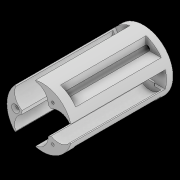
# Autodesk Inventor part: akkuhalterung_2
Saved by Autodesk Inventor 2022 (Build 260153000, 153)
## iProperties
Created: 2021-04-19
Part Number: akkuhalterung_2
Material: Generisch
Document SubType Name: Modeling
Designer: g.schardt
Density: 1 g/cm^3
Appearance: Vorgabe
Author: g.schardt
Autodesk Inventor part; units mm, degrees
ref_plane "YZ Plane" through (0, 0, 0) normal (1, 0, 0) x (0, 1, 0)
sketch "Skizze1" plane through (0, 0, 0) normal (0, 0, 1) x (1, 0, 0)
  circle A0 centre (0, 0) radius 20.25
  dimension "d0" = 40.5
  constraints: 1 centre point, 1 coincident
  measures "d0" diameter of A0
extrude "Extrusion1" add sketch "Skizze1" along normal blind 8
sketch "Skizze2" plane through (0, 0, 8) normal (0, 0, 1) x (1, 0, 0)
  circle A0 centre (11, 0) radius 9.5
  circle A1 centre (0, 0) radius 20.25 projected
  circle A2 centre (-5.5, 9.5263) radius 9.5
  circle A3 centre (-5.5, -9.5263) radius 9.5
  point P0 (1.5, 0)
  point P1 (-0.75, 1.299)
  point P2 (-0.75, -1.299)
  dimension "d3" = 19
  dimension "d6" = 360
  dimension "d251" = 40.5
  dimension "d252" = 11
  constraints: 3 horizontal alignment, 18 other
  measures "d251" diameter of A1
  measures "d252" distance of point (11, 0) A1.centre
extrude "Extrusion2" cut sketch "Skizze2" against normal blind 4.5 contours A0 A1 | A1 A0 | A2 A1 | A1 A2 | A3 A1 | A1 A3
sketch "Skizze3" plane through (-5.5, 9.5263, 8) normal (0, 0, 1) x (-0.8660254, -0.5, 0)
  circle A0 centre (0, 11) radius 10
  dimension "d10" = 20
  constraints: 1 centre point, 1 coincident
  measures "d10" diameter of A0
extrude "Extrusion3" cut sketch "Skizze3" against normal blind 4.5
sketch "Skizze4" plane through (0, 0, 3.5) normal (0, 0, 1) x (1, 0, 0)
  line L0 (5, 5.75) -> (25, 5.75)
  line L1 (25, 5.75) -> (25, -5.75)
  line L2 (25, -5.75) -> (5, -5.75)
  line L3 (5, -5.75) -> (5, 5.75)
  circle A0 centre (0, 0) radius 20.25 projected
  arc A1 (5.9432, -8.0423) -> (5.9432, 8.0423) centre (11, 0) ccw projected
  arc A2 (5.9432, 8.0423) -> (3.9932, 9.1681) centre (0, 0) ccw projected
  arc A3 (5.9432, -8.0423) -> (20.0369, -2.9298) centre (11, 0) ccw projected
  arc A4 (-7.4812, -18.8174) -> (20.0369, -2.9298) centre (0, 0) ccw projected
  arc A5 (3.9932, 9.1681) -> (-7.4812, 18.8174) centre (-5.5, 9.5263) ccw projected
  arc A6 (3.9932, -9.1681) -> (5.9432, -8.0423) centre (0, 0) ccw projected
  arc A7 (-9.9364, -1.1258) -> (-12.5558, -15.8876) centre (-5.5, -9.5263) ccw projected
  arc A8 (-9.9364, 1.1258) -> (-9.9364, -1.1258) centre (0, 0) ccw projected
  arc A9 (-12.5558, 15.8876) -> (-12.5558, -15.8876) centre (0, 0) ccw projected
  arc A10 (20.0369, 2.9298) -> (5.9432, 8.0423) centre (11, 0) ccw projected
  arc A11 (-12.5558, 15.8876) -> (-9.9364, 1.1258) centre (-5.5, 9.5263) ccw projected
  arc A12 (20.0369, 2.9298) -> (-7.4812, 18.8174) centre (0, 0) ccw projected
  arc A13 (-7.4812, -18.8174) -> (3.9932, -9.1681) centre (-5.5, -9.5263) ccw projected
  point P0 (25, 0)
  point P1 (20.25, 0)
  point P2 (19.4165, 5.75)
  point P3 (18.5622, 5.75)
  point P4 (19.4165, -5.75)
  point P5 (18.5622, -5.75)
  dimension "d13" = 20
  dimension "d14" = 11.5
  dimension "d33" = 6
  constraints: 8 end point, 2 parallel, 1 horizontal, 1 horizontal alignment, 1 midpoint, 1 perpendicular, 1 other
  measures "d13" distance of L1.end L2.end
  measures "d14" distance of L0.end L1.end
  measures "d33" distance from line of L3 A1.centre
extrude "Extrusion4" cut sketch "Skizze4" against normal blind 2 contours L0 A1 A0 L2 L3 | L0 A0 A1 | L0 L1 L2 A0 A1 | A1 A0 | A1 A0 L2
sketch "Skizze25" plane through (0, 0, 8) normal (0, 0, 1) x (1, 0, 0)
  arc A0 (19.4165, -5.75) -> (19.4165, 5.75) centre (0, 0) ccw projected
  line L0 (5, 5.75) -> (19.4165, 5.75) projected
  line L1 (5, -5.75) -> (5, 5.75) projected
  line L2 (19.4165, -5.75) -> (5, -5.75) projected
extrude "Extrusion21" cut sketch "Skizze25" against normal blind 4.5
sketch "Skizze6" plane through (0, 0, 3.5) normal (0, 0, 1) x (1, 0, 0)
  line L0 (5, 5.75) -> (14, 5.75)
  line L1 (14, 3.95) -> (5, 3.95)
  line L2 (5, 3.95) -> (5, 5.75)
  line L3 (18.5622, -5.75) -> (5, -5.75) projected
  line L4 (5, -5.75) -> (14, -5.75)
  line L5 (14, -3.95) -> (5, -3.95)
  line L6 (5, -3.95) -> (5, -5.75)
  line L7 (14, 3.95) -> (14, 5.75)
  line L8 (5, 5.75) -> (18.5622, 5.75) projected
  line L9 (14, -3.95) -> (14, -5.75)
  point P0 (0, 0)
  point P1 (19.4165, 5.75)
  point P2 (8.1815, -5.75)
  point P3 (8.1815, -5.75)
  dimension "d238" = 1.8
  dimension "d239" = 1.8
  dimension "d240" = 9
  dimension "d242" = 9
  constraints: 16 end point, 3 parallel, 2 horizontal, 2 perpendicular, 1 point on line
  measures "d238" distance of L1.end L0.start
  measures "d239" distance of L5.end L3.end
  measures "d240" distance of L1.start L1.end
  measures "d242" distance of L5.start L5.end
extrude "Extrusion6" add sketch "Skizze6" against normal blind 1.3
pattern_circular "Runde Anordnung1" count 3 over 360 about axis through (0, 0, 0) along (0, 0, 1) of "Extrusion4", "Extrusion6", "Extrusion21"
sketch "Skizze7" plane through (0, 0, 3.5) normal (0, 0, 1) x (1, 0, 0)
  circle A0 centre (0, 0) radius 5.5
  dimension "d40" = 11
  constraints: 1 centre point, 1 coincident
  measures "d40" diameter of A0
extrude "Extrusion7" cut sketch "Skizze7" against normal blind 2
sketch "Skizze26" plane through (0, 0, 8) normal (0, 0, 1) x (1, 0, 0)
  line L0 (-4.7286, 19.6902) -> (-4.3015, 18.9504) projected
  arc A0 (3.9932, 9.1681) -> (-4.3015, 18.9504) centre (-5.5, 9.5263) ccw projected
  arc A1 (5.9432, 8.0423) -> (3.9932, 9.1681) centre (0, 0) ccw projected
  arc A2 (18.5622, 5.75) -> (5.9432, 8.0423) centre (11, 0) ccw projected
  line L1 (18.5622, 5.75) -> (19.4165, 5.75) projected
  arc A3 (19.4165, 5.75) -> (-4.7286, 19.6902) centre (0, 0) ccw projected
  line L2 (-4.3015, -18.9504) -> (-4.7286, -19.6902) projected
  arc A4 (-4.7286, -19.6902) -> (19.4165, -5.75) centre (0, 0) ccw projected
  line L3 (19.4165, -5.75) -> (18.5622, -5.75) projected
  arc A5 (5.9432, -8.0423) -> (18.5622, -5.75) centre (11, 0) ccw projected
  arc A6 (3.9932, -9.1681) -> (5.9432, -8.0423) centre (0, 0) ccw projected
  arc A7 (-4.3015, -18.9504) -> (3.9932, -9.1681) centre (-5.5, -9.5263) ccw projected
  line L4 (-14.6879, -13.9402) -> (-14.2608, -13.2004) projected
  arc A8 (-9.9364, -1.1258) -> (-14.2608, -13.2004) centre (-5.5, -9.5263) ccw projected
  arc A9 (-9.9364, 1.1258) -> (-9.9364, -1.1258) centre (0, 0) ccw projected
  arc A10 (-14.2608, 13.2004) -> (-9.9364, 1.1258) centre (-5.5, 9.5263) ccw projected
  line L5 (-14.2608, 13.2004) -> (-14.6879, 13.9402) projected
  arc A11 (-14.6879, 13.9402) -> (-14.6879, -13.9402) centre (0, 0) ccw projected
extrude "Extrusion22" add sketch "Skizze26" along normal blind 58
sketch "Skizze28" plane through (0, 0, 0) normal (0, 0, -1) x (-1, 0, 0)
  circle A0 centre (0, 0) radius 14.8
  circle A1 centre (0, 0) radius 13.5
  dimension "d134" = 29.6
  dimension "d135" = 27
  constraints: 2 centre point, 2 coincident
  measures "d134" diameter of A0
  measures "d135" diameter of A1
extrude "Extrusion23" [suppressed]
sketch "Skizze29" plane through (0, 0, 66) normal (0, 0, 1) x (1, 0, 0)
  point P0 (0, 0)
  point P1 (-14.5, 0)
  dimension "d138" = 14.5
  constraints: 1 horizontal alignment
  measures "d138" distance of point (-14.5, 0) point (0, 0)
hole "Bohrung4" at (-14.5, 0, 66) direction (0, 0, -1) diameter 2.3 end through all
sketch "Skizze41" plane through (0, 0, 66) normal (0, 0, 1) x (1, 0, 0)
  circle A0 centre (-0.1, -0.1732) radius 2.5 construction
  circle A1 centre (-14.6, -0.1732) radius 1.75 construction
  circle A2 centre (-0.1, -0.1732) radius 14.5 construction
  line L0 (-0.1, -0.1732) -> (10.125, 17.537) construction
  circle A3 centre (0, 0) radius 20.25 construction
  line L1 (-0.1, -0.1732) -> (20.35, -0.1732) construction
  point P0 (7.15, 12.3842)
  dimension "d184" = 60
  constraints: 4 end point, 2 point on circle, 1 centre point, 1 coincident, 1 equal length, 1 horizontal, 1 point on line, 2 other
  measures "d184" angle of L1 L0
hole "Bohrung7" at (7.15, 12.3842, 66) direction (0, 0, -1) diameter 1.8 end through all
sketch "Skizze43" plane through (0, 0, 0) normal (0, 0, -1) x (-1, 0, 0)
  arc A0 (-8.0493, 12.4197) -> (-6.7311, 13.1807) centre (-7.15, 12.3842) ccw projected
  point P0 (0, 0)
hole "Bohrung8" at (7.15, 12.3842, 0) direction (0, 0, 1) diameter 3.5 depth 60 tip angle 118
pattern_circular "Runde Anordnung6" count 2 over 240 about axis through (0, 0, 0) along (0, 0, 1) of "Bohrung7", "Bohrung8"
sketch "Skizze44" plane through (0, 0, 0) normal (0, 0, -1) x (-1, 0, 0)
  circle A0 centre (0, 0) radius 20.25 projected
  circle A1 centre (0, 0) radius 18.25
  dimension "d202" = 2
  constraints: 1 centre point
  measures "d202" radial gap between concentric circles of A0 A1
extrude "Extrusion31" add sketch "Skizze44" along normal blind 3
sketch "Skizze45" plane through (0, 0, 1.5) normal (0, 0, 1) x (1, 0, 0)
  line L0 (0, 0) -> (-5, 8.6603) construction
  line L1 (0, 0) -> (10, 0) construction
  line L2 (0.9208, 6.3051) -> (-0.5157, 5.4758) construction
  point P0 (-1.25, 2.1651)
  dimension "d207" = 10
  dimension "d208" = 120
  dimension "d209" = 2.5
  constraints: 4 end point, 1 equal length, 1 horizontal, 1 point on line
  measures "d207" distance of L0.start L0.end
  measures "d208" angle of L1 L0
  measures "d209" distance from line of point (-1.25, 2.165) L2
hole "Bohrung9" at (-1.25, 2.1651, 1.5) direction (0, 0, -1) diameter 5 depth 80
sketch "Skizze46" plane through (0, 0, 66) normal (0, 0, 1) x (1, 0, 0)
  circle A0 centre (-14.5, 0) radius 1.15 projected
  arc A1 (-9.9364, 1.1258) -> (-9.9364, -1.1258) centre (0, 0) ccw projected
  arc A2 (-14.2608, 13.2004) -> (-9.9364, 1.1258) centre (-5.5, 9.5263) ccw projected
  line L0 (-14.2608, 13.2004) -> (-14.6879, 13.9402) projected
  arc A3 (-14.6879, 13.9402) -> (-14.6879, -13.9402) centre (0, 0) ccw projected
  line L1 (-14.6879, -13.9402) -> (-14.2608, -13.2004) projected
  arc A4 (-9.9364, -1.1258) -> (-14.2608, -13.2004) centre (-5.5, -9.5263) ccw projected
extrude "Extrusion32" add sketch "Skizze46" along normal blind 4
chamfer "Fase2" distance 1.5 angle 45 1 edges at (-15.65, 0, 70)
sketch "Skizze47" plane through (0, 0, 0) normal (0, 0, -1) x (-1, 0, 0)
  circle A0 centre (14.5, 0) radius 1.15 projected
  point P0 (0, 0)
hole "Bohrung10" at (-14.5, 0, 0) direction (0, 0, 1) diameter 3.5 depth 60 tip angle 118
ref_plane "Arbeitsebene4" through (0, 0, 60) normal (0, 0, 1) x (1, 0, 0)
sketch "Skizze48" plane through (0, 0, 60) normal (0, 0, 1) x (1, 0, 0)
  line L0 (6.25, 11.4842) -> (16.6786, 11.4842)
  line L1 (16.6786, 11.4842) -> (16.6786, 19.2614)
  line L2 (16.6786, 19.2614) -> (6.25, 19.2614)
  line L3 (6.25, 19.2614) -> (6.25, 11.4842)
  circle A0 centre (7.15, 12.3842) radius 0.9 projected
  circle A1 centre (0, 0) radius 20.25 projected
  point P0 (6.25, 12.3842)
  point P1 (7.15, 11.4842)
  constraints: 8 end point, 2 parallel, 2 point on circle, 2 tangent, 1 horizontal, 1 perpendicular
extrude "Extrusion33" cut sketch "Skizze48" against normal blind 58.5 contours A0 L3 A1 L0
ref_plane "Arbeitsebene5" through (0, 0, 60) normal (0, 0, 1) x (1, 0, 0)
sketch "Skizze49" plane through (0, 0, 60) normal (0, 0, 1) x (1, 0, 0)
  circle A0 centre (7.15, -12.3842) radius 0.9 projected
  line L0 (6.25, -11.4842) -> (16.6786, -11.4842)
  line L1 (16.6786, -11.4842) -> (16.6786, -19.2614)
  line L2 (16.6786, -19.2614) -> (6.25, -19.2614)
  line L3 (6.25, -19.2614) -> (6.25, -11.4842)
  arc A1 (-4.7286, -19.6902) -> (19.4165, -5.75) centre (0, 0) ccw projected
  point P0 (7.15, -11.4842)
  point P1 (6.25, -12.3842)
  constraints: 8 end point, 2 parallel, 2 point on circle, 2 tangent, 1 horizontal, 1 perpendicular
extrude "Extrusion34" cut sketch "Skizze49" against normal blind 58.5 contours A0 L0 A1 L3
chamfer "Fase3" distance 1 angle 45 6 edges at (14, 4.85, 2.2) (14, -4.85, 2.2) (-11.2002, -9.6994, 2.2) (-2.7998, -14.5494, 2.2) (-2.7998, 14.5494, 2.2) (-11.2002, 9.6994, 2.2)
sketch "Skizze39" plane through (0, 0, 66) normal (0, 0, 1) x (1, 0, 0)
  circle A0 centre (0, 0) radius 20.4
  constraints: 1 centre point, 1 coincident
sketch "Skizze31" plane through (0, 0, 66) normal (0, 0, 1) x (1, 0, 0)
  line L0 (-20.25, -5.5) -> (-17.25, -5.5)
  line L1 (-17.25, -5.5) -> (-17.25, 5.5)
  line L2 (-17.25, 5.5) -> (-20.25, 5.5)
  line L3 (-20.25, 5.5) -> (-20.25, -5.5)
  arc A0 (-14.6879, 13.9402) -> (-14.6879, -13.9402) centre (0, 0) ccw projected
  point P0 (-17.25, 0)
  point P1 (-19.6446, 5.5)
  point P2 (-19.6446, -5.5)
  dimension "d153" = 3
  dimension "d154" = 11
  constraints: 8 end point, 2 parallel, 1 horizontal, 1 horizontal alignment, 1 midpoint, 1 perpendicular, 1 tangent
  measures "d153" distance of L2.end L1.end
  measures "d154" distance of L1.end L0.end
sketch "Skizze32" plane through (-17.4, -5.5, 66) normal (-1, 0, 0) x (0, 0, 1)
  line L0 (-66, 11) -> (0, 11) projected
  line L1 (0, 0) -> (-66, 0) projected
  line L2 (-66, 9.5) -> (0, 9.5)
  line L3 (0, 1.5) -> (-66, 1.5)
  line L4 (0, 11) -> (0, 0) projected
  line L5 (-66, 0) -> (-66, 11) projected
  point P0 (-66, 5.5)
  dimension "d157" = 1.5
  dimension "d158" = 1.5
  constraints: 4 end point, 2 parallel
  measures "d157" distance between parallel lines of L0 L2
  measures "d158" distance between parallel lines of L1 L3
sketch "Skizze33" plane through (-17.4, -5.5, 0) normal (-1, 0, 0) x (0, 0, 1)
  line L0 (66, 1.5) -> (0, 1.5) projected
  line L1 (0, 0) -> (0, 1.5) projected
  line L2 (66, 0) -> (0, 0) projected
  line L3 (66, 1.5) -> (66, 0) projected
  line L4 (0, 9.5) -> (66, 9.5) projected
  line L5 (66, 11) -> (66, 9.5) projected
  line L6 (66, 11) -> (0, 11) projected
  line L7 (0, 9.5) -> (0, 11) projected
  line L8 (10, 9.5) -> (10, 11)
  line L9 (66, 11) -> (0, 11) projected
  line L10 (66, 1.5) -> (0, 1.5) projected
  line L11 (10, 1.5) -> (10, 0)
  point P0 (0, 5.5)
  dimension "d161" = 10
  constraints: 4 end point, 4 point on line, 2 perpendicular, 1 collinear
  measures "d161" distance between parallel lines of L7 L8
sketch "Skizze36" plane through (-19.6446, 5.5, 66) normal (0, -1, 0) x (1, 0, 0)
  line L0 (0, -66) -> (0, 0) projected
  line L1 (0, -50.4919) -> (1.2446, -50.4919)
  line L2 (1.2446, -50.4919) -> (1.2446, -44)
  line L3 (1.2446, -44) -> (0, -44)
  line L4 (0, -44) -> (0, -50.4919)
  line L5 (1.2446, -66) -> (1.2446, -56) projected
  line L6 (1.2446, -56) -> (2.2446, -56) projected
  point P0 (19.6446, -66)
  point P1 (0, -44)
  dimension "d165" = 12
  constraints: 8 end point, 2 parallel, 1 collinear, 1 horizontal, 1 perpendicular, 1 point on line
  measures "d165" distance between parallel lines of L6 L3
sketch "Skizze37" plane through (-19.6446, -5.5, 66) normal (0, 1, 0) x (1, 0, 0)
  line L0 (0, 0) -> (0, 66) projected
  line L1 (0, 26) -> (1.2446, 26)
  line L2 (1.2446, 26) -> (1.2446, 31)
  line L3 (1.2446, 31) -> (0, 31)
  line L4 (0, 31) -> (0, 26)
  line L5 (1.2446, 56) -> (1.2446, 66) projected
  line L6 (2.2446, 56) -> (1.2446, 56) projected
  point P0 (19.6446, 66)
  point P1 (0, 31)
  dimension "d168" = 25
  dimension "d169" = 5
  constraints: 8 end point, 2 parallel, 1 collinear, 1 horizontal, 1 perpendicular, 1 point on line
  measures "d168" distance between parallel lines of L6 L3
  measures "d169" distance of L1.end L2.end
sketch "Skizze38" plane through (-17.4, -5.5, 66) normal (-1, 0, 0) x (0, 0, 1)
  line L0 (0, 1.5) -> (-56, 1.5) projected
  line L1 (0, 0) -> (-56, 0) projected
  line L2 (0, 1.5) -> (-6, 1.5)
  line L3 (-6, 1.5) -> (-6, 0)
  line L4 (-6, 0) -> (0, 0)
  line L5 (0, 0) -> (0, 1.5)
  line L6 (-56, 0) -> (-56, 1.5) projected
  line L7 (-56, 9.5) -> (0, 9.5) projected
  line L8 (0, 11) -> (-6, 11)
  line L9 (-6, 11) -> (-6, 9.5)
  line L10 (-6, 9.5) -> (0, 9.5)
  line L11 (0, 9.5) -> (0, 11)
  point P0 (-66, 5.5)
  point P1 (-6, 1.5)
  dimension "d172" = 50
  constraints: 16 end point, 4 parallel, 2 horizontal, 2 perpendicular, 2 point on line
  measures "d172" distance between parallel lines of L6 L3
